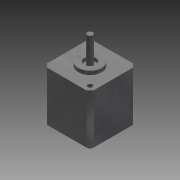
# Autodesk Inventor part: launcher_motor
Saved by Autodesk Inventor 2013 (Build 170138000, 138)
## iProperties
Created: 2013-07-24
Part Number: launcher_motor
Material: Generic
Document SubType Name: Modeling
Designer: dkboone
Density: 1 g/cm^3
Author: dkboone
Autodesk Inventor part; units mm, degrees
ref_plane "YZ Plane" through (0, 0, 0) normal (1, 0, 0) x (0, 1, 0)
ref_plane "XZ Plane" through (0, 0, 0) normal (0, 1, 0) x (-1, 0, 0)
ref_plane "XY Plane" through (0, 0, 0) normal (0, 0, 1) x (1, 0, 0)
sketch "Sketch1" plane through (0, 0, 0) normal (0, 1, 0) x (-1, 0, 0)
  line L0 (10.7, -12.7) -> (-10.7, -12.7)
  line L1 (-12.7, -10.7) -> (-12.7, 10.7)
  line L2 (-10.7, 12.7) -> (10.7, 12.7)
  line L3 (12.7, 10.7) -> (12.7, -10.7)
  line L4 (12.7, -10.7) -> (10.7, -12.7)
  line L5 (-10.7, -12.7) -> (-12.7, -10.7)
  line L6 (-12.7, 10.7) -> (-10.7, 12.7)
  line L7 (10.7, 12.7) -> (12.7, 10.7)
  circle A0 centre (9.525, -9.525) radius 1.27
  circle A1 centre (-9.525, 9.525) radius 1.27
  point P0 (0, 0)
  point P1 (12.7, -12.7)
  point P2 (-12.7, 12.7)
  point P3 (-12.7, -12.7)
  point P4 (12.7, 12.7)
  dimension "d0" = 25.4
  dimension "d2" = 25.4
  dimension "d3" = 12.7
  dimension "d4" = 12.7
  dimension "d5" = 2
  dimension "d6" = 2
  dimension "d7" = 2
  dimension "d8" = 2
  dimension "d9" = 2
  dimension "d10" = 2
  dimension "d11" = 2
  dimension "d12" = 2
  dimension "d13" = 3.175
  dimension "d14" = 3.175
  dimension "d15" = 3.175
  dimension "d16" = 3.175
  dimension "d17" = 2.54
  dimension "d18" = 2.54
  constraints: 16 end point, 8 point on line, 2 centre point, 2 parallel, 1 horizontal, 1 perpendicular
  measures "d0" distance between parallel lines of L1 L3
  measures "d2" distance of point (-12.7, -12.7) point (-12.7, 12.7)
  measures "d3" distance from line of point (0, 0) L0
  measures "d4" distance from line of point (0, 0) L1
  measures "d5" distance of L3.end point (12.7, -12.7)
  measures "d6" distance of L0.start point (12.7, -12.7)
  measures "d7" distance of L0.end point (-12.7, -12.7)
  measures "d8" distance of L1.start point (-12.7, -12.7)
  measures "d9" distance of L1.end point (-12.7, 12.7)
  measures "d10" distance of L2.start point (-12.7, 12.7)
  measures "d11" distance of L2.end point (12.7, 12.7)
  measures "d12" distance of L3.start point (12.7, 12.7)
  measures "d13" distance from line of L0 A0.centre
  measures "d14" distance from line of L3 A0.centre
  measures "d15" distance from line of L2 A1.centre
  measures "d16" distance from line of L1 A1.centre
  measures "d17" diameter of A0
  measures "d18" diameter of A1
extrude "Extrusion1" add sketch "Sketch1" along normal blind 26.9875
sketch "Sketch2" plane through (0, 26.9875, 0) normal (0, 1, 0) x (1, 0, 0)
  circle A0 centre (0, 0) radius 6.35
  circle A1 centre (0, 0) radius 3.175
  dimension "d21" = 12.7
  dimension "d23" = 6.35
  constraints: 2 centre point, 2 coincident
  measures "d21" diameter of A0
  measures "d23" diameter of A1
extrude "Extrusion2" add sketch "Sketch2" along normal blind 2
sketch "Sketch3" plane through (0, 26.9875, 0) normal (0, 1, 0) x (1, 0, 0)
  circle A0 centre (0, 0) radius 6.35 projected
  circle A1 centre (0, 0) radius 1.5
  dimension "d26" = 3
  constraints: 1 centre point, 1 coincident
  measures "d26" diameter of A1
extrude "Extrusion3" add sketch "Sketch3" along normal blind 15 contours A1
sketch "Sketch4" plane through (0, 0, 0) normal (0, -1, 0) x (1, 0, 0)
  circle A0 centre (0, 0) radius 1.5
  dimension "d30" = 3
  constraints: 1 centre point, 1 coincident
  measures "d30" diameter of A0
extrude "Extrusion4" add sketch "Sketch4" along normal blind 11.1125
sketch "Sketch5" plane through (0, 0, 0) normal (0, -1, 0) x (1, 0, 0)
  circle A0 centre (0, 0) radius 1.5 projected
  circle A1 centre (0, 9.525) radius 0.7937
  circle A2 centre (9.525, 0) radius 0.7937
  line L0 (0, 0) -> (0, 9.525) construction
  line L1 (0, 0) -> (9.525, 0) construction
  dimension "d34" = 9.525
  dimension "d35" = 9.525
  dimension "d36" = 1.5875
  dimension "d37" = 1.5875
  constraints: 4 end point, 2 centre point, 1 horizontal, 1 vertical
  measures "d34" distance of L0.end L0.start
  measures "d35" distance of L1.end L0.start
  measures "d36" diameter of A1
  measures "d37" diameter of A2
extrude "Extrusion5" add sketch "Sketch5" along normal blind 2.3813 contours A1 | A2
equation "\"d3\" = 0.5 * d2"
equation "\"d4\" = 0.5 * d0"
equation "\"d6\" = d5"
equation "\"d7\" = d5"
equation "\"d8\" = d7"
equation "\"d9\" = d5"
equation "\"d10\" = d9"
equation "\"d11\" = d5"
equation "\"d12\" = d11"
body "Solid1"
